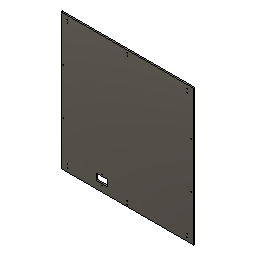
enclosure-back250 v10 (Autodesk Fusion 360 design; units mm, degrees)
Autodesk Fusion 360 part; units mm, degrees
sketch "Sketch1" plane through (0, 0, 0) normal (0, 0, 1) x (1, 0, 0)
  line L0 (284.2, -291.299) -> (-284.2, -291.299)
  line L1 (-284.2, -291.299) -> (-284.2, 291.299)
  line L2 (-284.2, 291.299) -> (284.2, 291.299)
  line L3 (284.2, 291.299) -> (284.2, -291.299)
  line L4 (284.2, -291.299) -> (-284.2, 291.299) construction
  line L5 (-284.2, -291.299) -> (284.2, 291.299) construction
  line L6 (-261.35, 291.299) -> (-261.35, -291.299) construction
  circle A0 centre (-261.35, 280.639) radius 2
  circle A1 centre (-261.35, 266.5) radius 2
  circle A2 centre (-261.35, -280.639) radius 2
  circle A3 centre (-261.35, -266.5) radius 2
  line L7 (261.35, 291.299) -> (261.35, -291.299) construction
  circle A4 centre (261.35, 280.639) radius 2
  circle A5 centre (261.35, 266.5) radius 2
  circle A6 centre (261.35, -280.639) radius 2
  circle A7 centre (261.35, -266.5) radius 2
  line L8 (-261.35, -266.5) -> (261.35, -266.5) construction
  circle A8 centre (0, -273.16) radius 2
  line L9 (0, -291.299) -> (0, 291.299) construction
  circle A9 centre (0, 273.16) radius 2
  circle A10 centre (0, 287.299) radius 2
  circle A11 centre (0, -287.299) radius 2
  line L10 (-289.2, 296.299) -> (289.2, 296.299)
  line L11 (289.2, 296.299) -> (289.2, -296.299)
  line L12 (289.2, -296.299) -> (-289.2, -296.299)
  line L13 (-289.2, -296.299) -> (-289.2, 296.299)
  line L14 (-289.2, -101.299) -> (289.2, -101.299) construction
  line L15 (-289.2, 101.299) -> (289.2, 101.299) construction
  circle A12 centre (-279.2, 101.299) radius 2
  circle A13 centre (-279.2, -101.299) radius 2
  circle A14 centre (279.2, -101.299) radius 2
  circle A15 centre (279.2, 101.299) radius 2
  line L16 (-134.2, -236.299) -> (-86.2, -236.299)
  line L17 (-86.2, -236.299) -> (-86.2, -263.799)
  line L18 (-86.2, -263.799) -> (-134.2, -263.799)
  line L19 (-134.2, -263.799) -> (-134.2, -236.299)
  line L20 (-110.2, -221.3553) -> (-110.2, -265.3735) construction
  circle A16 centre (-110.2, -270.549) radius 2
  circle A17 centre (-110.2, -229.549) radius 2
  line L21 (-261.35, 266.5) -> (261.35, 266.5) construction
  line L22 (-261.35, -280.639) -> (261.35, -280.639) construction
  line L23 (261.35, 280.639) -> (-261.35, 280.639) construction
  dimension "d1" = 568.4
  dimension "d2" = 582.598
  dimension "d3" = 22.85
  dimension "d4" = 4
  dimension "d6" = 4
  dimension "d8" = 4
  dimension "d9" = 4
  dimension "d12" = 22.85
  dimension "d13" = 4
  dimension "d14" = 4
  dimension "d17" = 4
  dimension "d18" = 4
  dimension "d21" = 4
  dimension "d22" = 4
  dimension "d23" = 4
  dimension "d24" = 4
  dimension "d30" = 5
  dimension "d31" = 5
  dimension "d32" = 5
  dimension "d33" = 5
  dimension "d34" = 190
  dimension "d35" = 190
  dimension "d36" = 4
  dimension "d37" = 5
  dimension "d38" = 4
  dimension "d39" = 5
  dimension "d40" = 4
  dimension "d41" = 5
  dimension "d42" = 4
  dimension "d43" = 5
  dimension "d44" = 48
  dimension "d45" = 27.5
  dimension "d46" = 55
  dimension "d47" = 150
  dimension "d48" = 24
  dimension "d49" = 4
  dimension "d50" = 4
  dimension "d51" = 41
  dimension "d52" = 20.5
  dimension "d53" = 24.799
  dimension "d54" = 24.799
  dimension "d55" = 10.66
  dimension "d56" = 10.66
  dimension "d60" = 14.139
  dimension "d61" = 4
  dimension "d62" = 14.139
  dimension "d63" = 4
  measures "d3" distance of L1 L6
  measures "d4" diameter of A0
  measures "d6" diameter of A1
  measures "d8" diameter of A2
  measures "d9" diameter of A3
  measures "d12" distance of L3 L7
  measures "d13" diameter of A4
  measures "d14" diameter of A5
  measures "d17" diameter of A6
  measures "d18" diameter of A7
  measures "d21" diameter of A8
  measures "d22" diameter of A9
  measures "d23" diameter of A10
  measures "d24" diameter of A11
  measures "d30" distance of L3 L11
  measures "d31" distance of L0 L12
  measures "d32" distance of L1 L13
  measures "d33" distance of L2 L10
  measures "d34" distance of L2 L15
  measures "d35" distance of L0 L14
  measures "d36" diameter of A12
  measures "d38" diameter of A13
  measures "d40" diameter of A14
  measures "d42" diameter of A15
  measures "d46" distance of L0 L16
  measures "d47" distance of L1 L19
  measures "d48" distance of L19 L20
  measures "d49" diameter of A16
  measures "d50" diameter of A17
  measures "d53" distance of L2 L21
  measures "d54" distance of L0 L8
  measures "d55" distance of L0 L22
  measures "d56" distance of L2 L23
extrude "Extrude1" add sketch "Sketch1" along normal blind 6.35 contours L0 L1 L2 L3 | L10 L11 L12 L13 makes body 1
copy_body "Body->Comp1" bodies 1 removing the originals makes body 2 in component "back"
component "back" placed x (1, 0, 0) y (0, 1, 0) z (0, 0, 1) at (0, 0, 0)
equation "d1 = XRailLength + 218.4 mm"
equation "d2 = PrintHeight + 282.598 mm"
equation "d28 = ( 25.4 / 4 ) * 1 mm"
equation "d30 = WallThickness"
equation "d31 = WallThickness"
equation "d32 = WallThickness"
equation "d33 = WallThickness"
equation "WallThickness = 5 mm"
equation "XRailLength = 350 mm"
equation "PrintHeight = 300 mm"
named bodies: "back"
